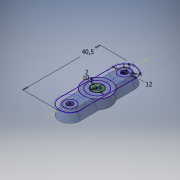
# Autodesk Inventor part: HarmonicDrive-WaveGenerator-Bottom
Saved by Autodesk Inventor 2018.3 (Build 223284000, 284)
## iProperties
Created: 2018-06-23
Part Number: HarmonicDrive-WaveGenerator-Bottom
Material: Generisch
Document SubType Name: Modeling
Designer: JochenAlt
Density: 1 g/cm^3
Appearance: Gummi - blau
Author: JochenAlt
Autodesk Inventor part; units mm, degrees
ref_plane "YZ Plane" through (0, 0, 0) normal (1, 0, 0) x (0, 1, 0)
ref_plane "XZ Plane" through (0, 0, 0) normal (0, 1, 0) x (-1, 0, 0)
ref_plane "XY Plane" through (0, 0, 0) normal (0, 0, 1) x (1, 0, 0)
sketch "Skizze1" plane through (0, 0, 0) normal (0, 0, 1) x (1, 0, 0)
  line L0 (0, -14.25) -> (0, 14.25) construction
  line L1 (5.5, -14.25) -> (5.5, 14.25)
  line L2 (-5.5, 14.25) -> (-5.5, -14.25)
  arc A0 (-5.5, -14.25) -> (5.5, -14.25) centre (0, -14.25) ccw
  arc A1 (5.5, 14.25) -> (-5.5, 14.25) centre (0, 14.25) ccw
  line L3 (0, 28.35) -> (0, -28.35) construction
  line L4 (-9.8, 0) -> (9.8, 0) construction
  circle A2 centre (0, 14.25) radius 1.5
  circle A3 centre (0, -14.25) radius 1.5
  circle A4 centre (0, 0) radius 3
  circle A5 centre (0, 14.25) radius 6 construction
  circle A6 centre (0, -14.25) radius 6 construction
  line L5 (0, 20.25) -> (0, -20.25) construction
  circle A7 centre (0, 14.25) radius 3
  circle A8 centre (0, -14.25) radius 3
  circle A9 centre (0, 0) radius 2.1461
  circle A10 centre (0, 0) radius 5
  circle A11 centre (0, 0) radius 7
  dimension "d4" = 12
  dimension "d1" = 3
  dimension "d2" = 4
  dimension "d3" = 6
  dimension "d5" = 40.5
  dimension "d19" = 1.5
  dimension "d22" = 10
  dimension "d23" = 2
  constraints: 10 centre point, 10 coincident, 10 end point, 4 point on circle, 4 tangent, 2 equal radius, 2 point on line, 2 vertical alignment, 1 midpoint, 1 parallel, 1 vertical, 4 other
  measures "d1" diameter of A2
  measures "d2" radial gap between concentric circles of A1 A2
  measures "d3" diameter of A4
  measures "d5" distance of L5.start L5.end
  measures "d19" radial gap between concentric circles of A2 A7
  measures "d22" diameter of A10
  measures "d23" radial gap between concentric circles of A11 A10
extrude "Extrusion1" add sketch "Skizze1" against normal blind 5 contours A0 L2 A11 L1 | A11 L2 L1 | L1 A11 | A11 L2 A1 L1 | A11 L2 | A7 | A8 | A10
chamfer "Fase2" distance 2 distance2 5 6 edges at (5.5, -9.2901, 0) (5.5, 9.2901, 0) (0, 19.75, 0) (-5.5, 9.2901, 0) (-5.5, -9.2901, 0) (0, -19.75, 0) measured on face at (0, 19.25, 0) measured on face at (-5, -9.2901, 0) measured on face at (5, 9.2901, 0) measured on face at (-5, 9.2901, 0) measured on face at (5, -9.2901, 0) measured on face at (0, -19.25, 0)
extrude "Extrusion4" add sketch "Skizze1" against normal blind 0.5 from surface at -5 contours A7 | A8
